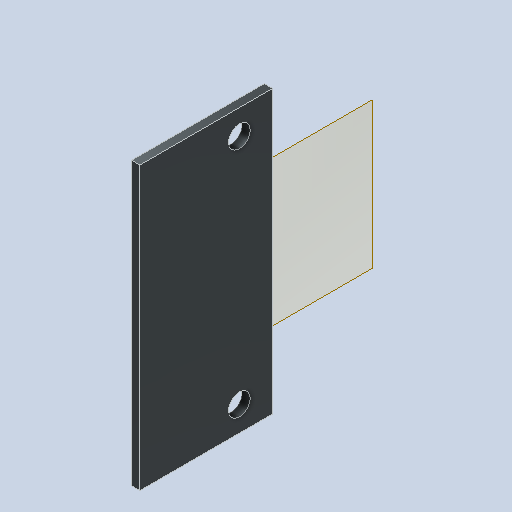
# Autodesk Inventor part: class3
Saved by Autodesk Inventor 2025.2 (Build 292293000, 293)
## iProperties
Created: 2024-07-24
Part Number: class3
Material: Iron, Ductile
Document SubType Name: Modeling
Designer: eamon
Density: 7.15 g/cm^3
Appearance: Iron Gray
Author: eamon
Autodesk Inventor part; units mm, degrees
ref_plane "YZ Plane" through (0, 0, 0) normal (1, 0, 0) x (0, 1, 0)
ref_plane "XZ Plane" through (0, 0, 0) normal (0, 1, 0) x (-1, 0, 0)
ref_plane "XY Plane" through (0, 0, 0) normal (0, 0, 1) x (1, 0, 0)
ref_plane "Work Plane1" through (178.2845, 12.3881, -65.7398) normal (1, 0, 0) x (0, 1, 0)
sketch "Sketch1" plane through (178.2845, 12.3881, -65.7398) normal (1, 0, 0) x (0, 1, 0)
  line L0 (57.15, 50.8) -> (-158.75, 50.8)
  line L1 (-158.75, 50.8) -> (-158.75, -50.8)
  line L2 (-158.75, -50.8) -> (57.15, -50.8)
  line L3 (57.15, -50.8) -> (57.15, 50.8)
  line L4 (63.5, -127) -> (-165.1, -127) construction
  line L5 (19.05, 0) -> (19.05, -127) construction
  circle A0 centre (38.1, -25.4) radius 8.255
  circle A1 centre (-139.7, -25.4) radius 8.255
  point P0 (-12.3881, 65.7398)
  point P1 (-50.8, -127)
  point P2 (-50.8, -50.8)
  point P3 (57.15, 0)
  dimension "d0" = 101.6
  dimension "d1" = 215.9
  dimension "d2" = 16.51
  dimension "d3" = 177.8
  dimension "d4" = 19.05
  dimension "d5" = 25.4
  constraints: 8 end point, 3 midpoint, 2 centre point, 2 horizontal alignment, 2 parallel, 1 equal radius, 1 horizontal, 1 perpendicular, 1 vertical alignment
  measures "d0" distance of L2.end L0.start
  measures "d1" distance of L0.start L0.end
  measures "d2" diameter of A0
  measures "d3" distance of A1.centre A0.centre
  measures "d4" distance from line of L3 A0.centre
  measures "d5" distance from line of L2 A0.centre
extrude "Extrusion1" add sketch "Sketch1" along normal blind 6.35
body "Solid1"
